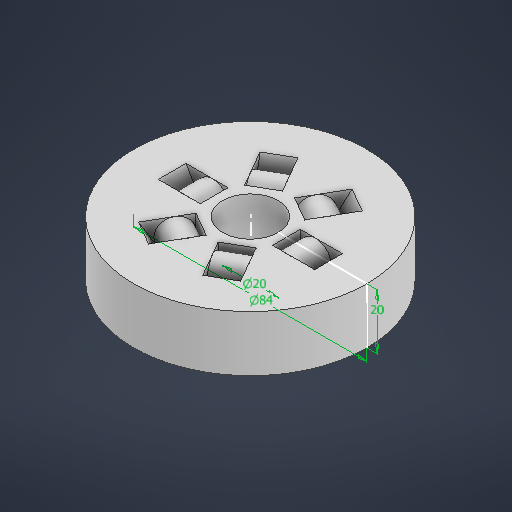
# Autodesk Inventor part: self-regulating
Saved by Autodesk Inventor 2026.2 (Build 302298000, 298)
## iProperties
Created: 2026-01-20
Part Number: self-regulating
Material: 一般
Document SubType Name: Modeling
Designer: JustA
Density: 1 g/cm^3
Appearance: 預設
Author: JustA
Autodesk Inventor part; units mm, degrees
ref_plane "YZ Plane" through (0, 0, 0) normal (1, 0, 0) x (0, 1, 0)
ref_plane "XZ Plane" through (0, 0, 0) normal (0, 1, 0) x (-1, 0, 0)
ref_plane "XY Plane" through (0, 0, 0) normal (0, 0, 1) x (1, 0, 0)
sketch "草圖1" plane through (0, 0, 0) normal (0, 0, 1) x (1, 0, 0)
  line L0 (0, -12.1345) -> (0, 12.1345)
  line L1 (10, -10) -> (42, -10)
  line L2 (42, -10) -> (42, 10)
  line L3 (42, 10) -> (10, 10)
  line L4 (10, 10) -> (10, -10)
  line L5 (-15.5263, 0) -> (15.5263, 0)
  point P0 (0, 0)
  point P1 (0, 0)
  point P2 (10, 0)
  dimension "d0" = 20
  dimension "d1" = 20
  dimension "d2" = 84
  constraints: 12 end point, 3 midpoint, 2 horizontal, 2 parallel, 1 coincident, 1 perpendicular, 1 point on line, 1 vertical
  measures "d0" diameter of L4 L0
  measures "d1" distance of L1.end L2.end
  measures "d2" diameter of L2 L0
revolve "迴轉1" add sketch "草圖1" angle 360 about axis through (0, -12.1345, 0) along (0, 1, 0)
sketch "草圖3" plane through (0, 0, 0) normal (0, 0, 1) x (1, 0, 0)
  line L0 (42, 10) -> (10, 10) projected
  line L1 (-15.5263, 0) -> (15.5263, 0) projected
  circle A0 centre (18.5574, 4.4426) radius 5.5574
  line L2 (28.183, 10) -> (21.7659, -1.1147)
  line L3 (21.7659, -1.1147) -> (13, -1.1147)
  line L4 (10, 10) -> (10, -10) projected
  line L5 (13, 10) -> (13, -1.1147)
  point P0 (0, 0)
  dimension "d5" = 60
  dimension "d6" = 3
  constraints: 6 end point, 4 tangent, 2 point on line, 1 centre point, 1 horizontal, 1 perpendicular
  measures "d5" angle of L3 L2
  measures "d6" distance between parallel lines of L4 L5
extrude "擠出1" cut sketch "草圖3" along normal mid plane 10 contours L0 A0 L5 | L0 L2 A0 | A0 | A0 L1 L5 | A0 L3 L5 L1 | L2 L3 A0
pattern_circular "環形陣列1" count 6 over 360 about axis through (0, -10, 0) along (0, 1, 0) of "擠出1"
sketch "草圖4" plane through (0, 10, 0) normal (0, 1, 0) x (1, 0, 0)
  line L0 (0, 12.7017) -> (11, 6.3509)
  line L1 (11, 6.3509) -> (11, -6.3509)
  line L2 (11, -6.3509) -> (0, -12.7017)
  line L3 (0, -12.7017) -> (-11, -6.3509)
  line L4 (-11, -6.3509) -> (-11, 6.3509)
  line L5 (-11, 6.3509) -> (0, 12.7017)
  line L6 (13, -5) -> (13, 5) projected
  point P0 (0, 0)
  point P1 (0, 0)
  dimension "d12" = 11
  dimension "d13" = 2
  constraints: 12 end point, 1 coincident, 13 other
  measures "d12" distance from line of L1 point (0, 0)
  measures "d13" distance between parallel lines of L6 L1
extrude "擠出2" add sketch "草圖3" along normal mid plane 10 separate body contours A0
pattern_circular "環形陣列2" count 6 over 360 about axis through (0, -10, 0) along (0, 1, 0) of "擠出2" bodies 2
